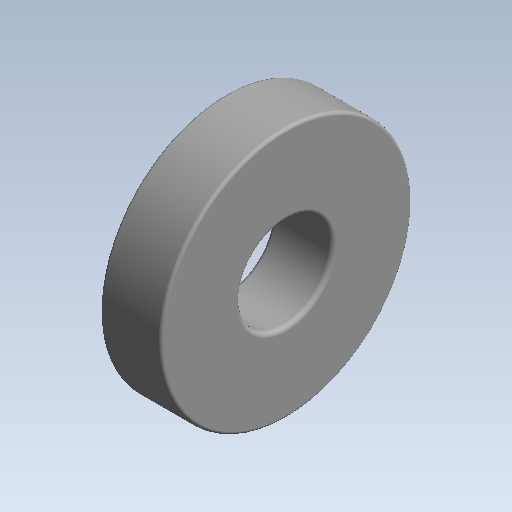
# Autodesk Inventor part: 110202DT-20-L1260ZZ_ball
Saved by Autodesk Inventor 2021.3 (Build 253353010, 353A)
## iProperties
Part Number: 110202DT-20-L1260ZZ_ball
Material: 一般
Catalog Web Link: www.cadenas.de
Description: DT ball-I-Series bearings
Vendor: TOKBEARING
Document SubType Name: Modeling
Designer: partserver
Manufacturer: TOKBEARING
Mass: 0.730338 g
Surface Area: 6.34078 cm^2
Volume: 0.730338 cm^3
Density: 1 g/cm^3
Appearance: PSOLRGB-192-192-192
Category: PARTsolutions
Company: TOKBEARING
PSOL_IDENT_0: {$CADENAS_DATA\23d-libs\tok_bearing\i_series_bearings\dt\dt_ball.prj},191 {VTYP=3D},{NB=110202DT-20-
PSOL_IDENT_1: L1260ZZ_ball},{LINA=110202DT-20-L1260ZZ_ball},{NN=DT ball},{DATE=16.12.2020 00:38:07},{GEOMDATE=31.0
PSOL_IDENT_2: 7.2014 05:09:00},{VERSION=},{LINEID=2930},{WBVAR=},{WBNUMERIC=}  {NB=110202DT-20-L1260ZZ_ball},{LINA=
PSOL_IDENT_3: 110202DT-20-L1260ZZ_ball},{KT=DUMMY},{IDNR=},{CODE=110202},{PN=DT-20-L1260ZZ},{D=20},{SD=6},{SDX=6.0
PSOL_IDENT_4: 00},{W=6},{C=-},{CX=0.000},{L=-},{LX=0.000},{N=-},{NX=0.000},{TYPE=1},{B=4},{BD=4},{OP=35.168},{BQ=5
PSOL_IDENT_5: },{R=5.6},{GP=2.4}
NB: 110202DT-20-L1260ZZ_ball
NN: DT ball
NT: I-Series bearings
NBSYN: $CODE.$PN._ball
LINA: 110202DT-20-L1260ZZ_ball
CATALOG: TOK, Inc
CODE: 110202
PN: DT-20-L1260ZZ
D: 20
SD: 6
SDX: 6
W: 6
C: -
CX: 0
L: -
LX: 0
N: -
NX: 0
TYPE: 1
B: 4
SUPPLIER: TOKBEARING
ARTICLENO: 110202DT-20-L1260ZZ_ball
BOMINFO: 110202DT-20-L1260ZZ_ball
CREATOR: CADENAS GmbH
Title: 110202DT-20-L1260ZZ_ball
Author: Cadenas PARTsolutions
Comments: I-Series bearings
Autodesk Inventor part; units mm, degrees
sketch "Sketch_4" plane through (0, 0, 0) normal (0, 0, 1) x (1, 0, 0)
  line L0 (50, 0) -> (-50, 0)
  arc A0 (-2, 3.28) -> (-1.72, 3) centre (-1.72, 3.28) ccw
  line L1 (-1.72, 3) -> (1.72, 3)
  arc A1 (1.72, 3) -> (2, 3.28) centre (1.72, 3.28) ccw
  line L2 (2, 3.28) -> (2, 8)
  arc A2 (2, 8) -> (1.8, 8.2) centre (1.8, 8) ccw
  line L3 (1.8, 8.2) -> (-1.8, 8.2)
  arc A3 (-1.8, 8.2) -> (-2, 8) centre (-1.8, 8) ccw
  line L4 (-2, 8) -> (-2, 3.28)
  constraints: 10 end point, 8 point on circle, 4 centre point
revolve "Revolution1" add sketch "Sketch_4" angle 360 about axis through (50, 0, 0) along (1, 0, 0)
ref_plane "IP_ball_XY" through (0, 0, 0) normal (1, 0, 0) x (0, 0, -1)
ref_plane "IP_ball_YZ" through (0, 0, 0) normal (0, 0, -1) x (0, 1, 0)
ref_plane "IP_ball_ZX" through (0, 0, 0) normal (0, 1, 0) x (1, 0, 0)
body "Solid1"
